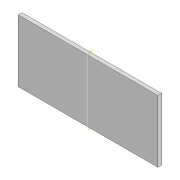
# Autodesk Inventor part: new_wire_bottom
Saved by Autodesk Inventor 2020 (Build 240168000, 168)
## iProperties
Created: 2021-05-13
Part Number: new_wire_bottom
Material: Generic
Document SubType Name: Modeling
Designer: Hsu Daniel
Density: 1 g/cm^3
Appearance: Default
Author: Hsu Daniel
Autodesk Inventor part; units mm, degrees
ref_plane "YZ Plane" through (0, 0, 0) normal (1, 0, 0) x (0, 1, 0)
ref_plane "XZ Plane" through (0, 0, 0) normal (0, 1, 0) x (-1, 0, 0)
ref_plane "XY Plane" through (0, 0, 0) normal (0, 0, 1) x (1, 0, 0)
sketch "Sketch1" plane through (0, 0, 0) normal (0, 0, 1) x (1, 0, 0)
  line L0 (0, 0) -> (202, 0)
  line L1 (202, 0) -> (202, 90)
  line L2 (202, 90) -> (0, 90)
  line L3 (0, 90) -> (0, 0)
  dimension "d3" = 202
  dimension "d4" = 90
  constraints: 8 end point, 2 parallel, 1 horizontal, 1 perpendicular
  measures "d3" distance of L1.end L2.end
  measures "d4" distance of L0.end L1.end
extrude "Extrusion1" add sketch "Sketch1" along normal blind 5.5
ref_plane "Work Plane1" through (101, 0, 0) normal (1, 0, 0) x (0, 0, -1)
equation "\"thick\" = 0.5"
equation "\"lrlr\" = 19"
equation "\"lrmid\" = 19.9"
equation "\"lrdepth\" = 3.3"
equation "\"mlr\" = 16.6"
equation "\"mmid\" = 24.7"
equation "\"mdepth\" = 4.5"
equation "\"lrltotal\" = 126.6"
equation "\"mltotal\" = 126.6"
equation "\"lrbetween\" = 52.1"
equation "\"mbetween\" = 49.5"
equation "\"toler\" = 1"
equation "\"tight\" = 0.08"
equation "\"stuckw\" = 6"
equation "\"sidewallL\" = 132.6"
equation "\"heaterH\" = 117.3"
equation "\"stickL\" = 3.5"
equation "\"wireH\" = 25"
body "Solid1"
